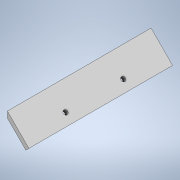
# Autodesk Inventor part: nozyk
Saved by Autodesk Inventor 2022 (Build 260153000, 153)
## iProperties
Created: 2022-12-25
Part Number: nozyk
Material: Generic
Document SubType Name: Modeling
Designer: Kamil
Density: 1 g/cm^3
Appearance: Default
Author: Kamil
Autodesk Inventor part; units mm, degrees
ref_plane "YZ Plane" through (0, 0, 0) normal (1, 0, 0) x (0, 1, 0)
ref_plane "XZ Plane" through (0, 0, 0) normal (0, 1, 0) x (-1, 0, 0)
ref_plane "XY Plane" through (0, 0, 0) normal (0, 0, 1) x (1, 0, 0)
sketch "Sketch1" plane through (0, 0, 0) normal (0, 0, 1) x (1, 0, 0)
  line L0 (0, 50.1071) -> (-7.1, 57.2071) projected
  line L1 (-7.1, 57.2071) -> (-7.1, 0) projected
  line L2 (0, 0) -> (-7.1, 0) projected
  line L3 (0, 50.1071) -> (0, 0) projected
  circle A0 centre (6, -18.6) radius 16.1 projected
  line L4 (-10.1, -18.6) -> (-10.1, 64.4833)
  line L5 (-7.1, 57.2071) -> (-10.1, 60.2071)
  line L6 (-10.1, 60.2071) -> (2.6279, 47.4792)
  line L7 (2.6279, 47.4792) -> (4.7492, 49.6005)
  line L8 (4.7492, 49.6005) -> (-14.184, 68.5338)
  line L9 (-10.1, 64.4833) -> (-10.1, 67.3257)
  point P0 (-10.1, 64.4498)
  dimension "d0" = 18
  dimension "d1" = 3
  constraints: 12 end point, 2 point on line, 2 vertical, 1 horizontal alignment, 1 parallel, 1 other
  measures "d0" distance of L6.start L6.end
  measures "d1" distance of L6.end L7.end
ref_plane "Work Plane1" through (-7.1, 0, -96) normal (0, 0, -1) x (0, 1, 0)
extrude "Extrusion1" add sketch "Sketch1" against normal up to surface (96 mm away) contours L0 L5 L4 L8 L7 L6
sketch "Sketch2" plane through (-10.1, 64.4498, -96) normal (0.7071068, 0.7071068, 0) x (-0.7071068, 0.7071068, 0)
  circle A0 centre (-14.7131, 28.1488) radius 1.5 projected
  circle A1 centre (-14.7131, 67.8512) radius 1.5 projected
  point P0 (-52.7147, 96)
extrude "Extrusion2" cut sketch "Sketch2" against normal through all
sketch "Sketch3" plane through (-10.1, 60.2071, -96) normal (0, 0, -1) x (-1, 0, 0)
  line L0 (0, 4.2426) -> (0, 0) projected
  line L1 (-14.8492, -10.6066) -> (0, 4.2426) projected
  line L2 (-12.7279, -12.7279) -> (-14.8492, -10.6066) projected
  line L3 (0, 0) -> (-12.7279, -12.7279) projected
  point P0 (-10.1, -60.2071)
ref_plane "Work Plane2" through (-7.1, -33.8, -97.5) normal (0, 0, -1) x (0, 1, 0)
extrude "Extrusion3" add sketch "Sketch3" along normal up to surface (1.5 mm away)
sketch "Sketch4" plane through (0, 0, 0) normal (0, 0, 1) x (1, 0, 0)
  line L0 (4.7492, 49.6005) -> (-10.1, 64.4498) projected
  line L1 (-10.1, 64.4498) -> (-10.1, 60.2071) projected
  line L2 (-10.1, 60.2071) -> (2.6279, 47.4792) projected
  line L3 (2.6279, 47.4792) -> (4.7492, 49.6005) projected
  point P0 (0, 0)
ref_plane "Work Plane3" through (-7.1, -33.8, 1.5) normal (0, 0, 1) x (1, 0, 0)
extrude "Extrusion4" add sketch "Sketch4" along normal up to surface (1.5 mm away)
body "Solid1"
